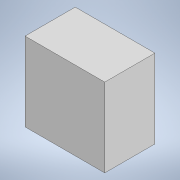
# Autodesk Inventor part: Heatsink
Saved by Autodesk Inventor 2021 (Build 250183000, 183)
## iProperties
Created: 2020-10-20
Part Number: Heatsink
Material: Generic
Document SubType Name: Modeling
Designer: VM
Density: 1 g/cm^3
Appearance: Default
Author: VM
Autodesk Inventor part; units mm, degrees
ref_plane "YZ Plane" through (0, 0, 0) normal (1, 0, 0) x (0, 1, 0)
ref_plane "XZ Plane" through (0, 0, 0) normal (0, 1, 0) x (-1, 0, 0)
ref_plane "XY Plane" through (0, 0, 0) normal (0, 0, 1) x (1, 0, 0)
sketch "Sketch1" plane through (0, 0, 0) normal (0, 0, 1) x (1, 0, 0)
  line L0 (0, 0) -> (37.8, 0)
  line L1 (37.8, 0) -> (37.8, -37.3)
  line L2 (37.8, -37.3) -> (0, -37.3)
  line L3 (0, -37.3) -> (0, 0)
  dimension "d0" = 37.8
  dimension "d1" = 37.3
  constraints: 8 end point, 2 parallel, 1 horizontal, 1 perpendicular
  measures "d0" distance of L1.end L2.end
  measures "d1" distance of L0.end L1.end
extrude "Extrusion1" add sketch "Sketch1" along normal blind 23.8
body "Solid1"
